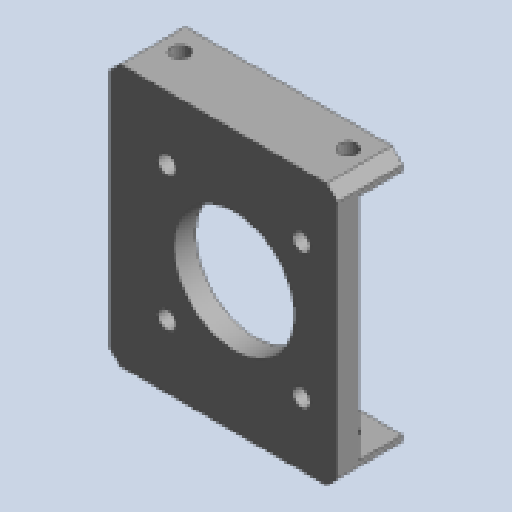
# Autodesk Inventor part: MotorMount
Saved by Autodesk Inventor 2023 (Build 270158000, 158)
## iProperties
Created: 2024-02-25
Part Number: MotorMount
Material: Generic
Document SubType Name: Modeling
Designer: valer
Density: 1 g/cm^3
Appearance: Default
Author: valer
Autodesk Inventor part; units mm, degrees
ref_plane "YZ Plane" through (0, 0, 0) normal (1, 0, 0) x (0, 1, 0)
ref_plane "XZ Plane" through (0, 0, 0) normal (0, 1, 0) x (-1, 0, 0)
sketch "Base" plane through (0, 0, 0) normal (0, 0, 1) x (1, 0, 0)
  circle A0 centre (0, 0) radius 11 construction
  line L0 (18, 21) -> (-22, 21) construction
  line L1 (-22, -21) -> (18, -21) construction
  line L2 (19, -20) -> (19, 20) construction
  line L3 (-23, 20) -> (-23, -20) construction
  circle A1 centre (0, 0) radius 11.075
  line L4 (-197.84, 0) -> (55.14, 0) construction
  line L5 (-23, 23.05) -> (19, 23.05)
  line L6 (19, 23.05) -> (19, 21.05)
  line L7 (19, 21.05) -> (-23, 21.05)
  line L8 (-23, 21.05) -> (-23, 23.05)
  line L9 (-23, 21.05) -> (19, 21.05)
  line L10 (19, 21.05) -> (19, 0)
  line L11 (19, 0) -> (-23, 0)
  line L12 (-23, 0) -> (-23, 21.05)
  line L13 (-23, -23.05) -> (19, -23.05)
  line L14 (19, -23.05) -> (19, -21.05)
  line L15 (19, -21.05) -> (-23, -21.05)
  line L16 (-23, -21.05) -> (-23, -23.05)
  line L17 (19, -21.05) -> (19, 0)
  line L18 (-23, 0) -> (-23, -21.05)
  line L19 (0, 14) -> (0, 0) construction
  line L20 (0, 0) -> (0, -14) construction
  circle A2 centre (12.3744, -12.3744) radius 1.621 projected
  circle A3 centre (12.3744, 12.3744) radius 1.621 projected
  circle A4 centre (-12.3744, 12.3744) radius 1.621 projected
  circle A5 centre (-12.3744, -12.3744) radius 1.621 projected
  dimension "d0" = 22.15
  dimension "d1" = 2
  dimension "d4" = 0.05
  constraints: 34 end point, 5 symmetric about line, 4 parallel, 3 collinear, 3 perpendicular, 2 coincident, 2 horizontal, 1 centre point, 1 midpoint, 1 point on line, 1 vertical, 2 other
  measures "d0" diameter of A1
  measures "d1" distance of L5.end L6.end
  measures "d4" distance between parallel lines of L7 L0
extrude "BaseFeature" add sketch "Base" along normal blind 4 contours L11 L17 L15 L18 A1 | A1 L11 L12 L7 L10 | L7 L8 L5 L6 | L14 L13 L16 L15
ref_plane "Work Plane1" through (-20.5858, -18.5858, -56) normal (0, 0, -1) x (0, 1, 0)
sketch "Sides" plane through (0, 0, 0) normal (0, 0, -1) x (-1, 0, 0)
  line L0 (23, -23.05) -> (-19, -23.05) projected
  line L1 (-19, -23.05) -> (23, -23.05)
  line L2 (23, -23.05) -> (23, -21.05)
  line L3 (23, -21.05) -> (-19, -21.05)
  line L4 (-19, -21.05) -> (-19, -23.05)
  line L5 (-19, 23.05) -> (23, 23.05) projected
  line L6 (-19, 23.05) -> (23, 23.05)
  line L7 (23, 23.05) -> (23, 21.05)
  line L8 (23, 21.05) -> (-19, 21.05)
  line L9 (-19, 21.05) -> (-19, 23.05)
  point P0 (0, 0)
  constraints: 16 end point, 4 parallel, 2 horizontal, 2 perpendicular, 1 coincident
extrude "Extrusion2" add sketch "Sides" along normal blind 8
sketch "Sketch3" plane through (-23, -23.05, 4) normal (0, -1, 0) x (1, 0, 0)
  line L0 (42, -12) -> (42, 0) projected
  line L1 (0, 0) -> (42, 0) projected
  line L2 (0, -12) -> (0, 0) projected
  line L3 (42, -12) -> (0, -12) projected
  point P0 (23, -4)
extrude "Extrusion3" add sketch "Sketch3" along normal blind 1
mirror "Mirror1" about plane through (0, 0, 0) normal (0, 1, 0) of "Extrusion3"
sketch "Sketch4" plane through (-23, -24.05, 4) normal (0, -1, 0) x (1, 0, 0)
  line L0 (0, 0) -> (0, -12) construction
  line L1 (42, -4) -> (42, -12) construction
  circle A0 centre (5.5, -7.5) radius 1.621
  line L2 (21, 0) -> (21, -12) construction
  line L3 (0, -12) -> (42, -12) construction
  line L4 (42, 0) -> (0, 0) construction
  circle A1 centre (36.5, -7.5) radius 1.621
  point P0 (23, -4)
  dimension "d9" = 3.242
  dimension "d15" = 5.5
  dimension "d16" = 4.5
  constraints: 2 centre point, 2 end point, 2 midpoint, 1 perpendicular, 1 symmetric about line, 1 other
  measures "d9" diameter of A0
  measures "d15" distance from line of L0 A0.centre
  measures "d16" distance from line of L3 A0.centre
extrude "Extrusion4" cut sketch "Sketch4" against normal through all
chamfer "Chamfer1" distance 2 angle 45 4 edges at (19, 24.05, -2) (-23, 24.05, -2) (19, -24.05, -2) (-23, -24.05, -2)
body "Solid1"
